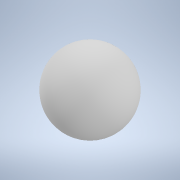
# Autodesk Inventor part: 9mm_ballbearing
Saved by Autodesk Inventor 2022 (Build 260153000, 153)
## iProperties
Created: 2022-03-14
Part Number: 9mm_ballbearing
Material: Generic
Document SubType Name: Modeling
Designer: Jorian Brusind
Density: 1 g/cm^3
Appearance: Default
Author: Jorian Brusind
Autodesk Inventor part; units mm, degrees
ref_plane "YZ Plane" through (0, 0, 0) normal (1, 0, 0) x (0, 1, 0)
ref_plane "XZ Plane" through (0, 0, 0) normal (0, 1, 0) x (-1, 0, 0)
ref_plane "XY Plane" through (0, 0, 0) normal (0, 0, 1) x (1, 0, 0)
sketch "Sketch1" plane through (0, 0, 0) normal (0, 1, 0) x (-1, 0, 0)
  arc A0 (-9, 0) -> (9, 0) centre (0, 0) ccw
  line L0 (0, 0) -> (-9, 0) construction
  line L1 (0, 0) -> (9, 0) construction
  line L2 (-9, 0) -> (9, 0)
  dimension "d0" = 9
  dimension "d1" = 180
  constraints: 6 end point, 2 point on circle, 1 centre point, 1 coincident, 1 horizontal
  measures "d0" radius of A0
  measures "d1" angle of L0 L1
revolve "Revolution1" add sketch "Sketch1" angle 360 about axis through (9, 0, 0) along (-1, 0, 0)
body "Solid1"
